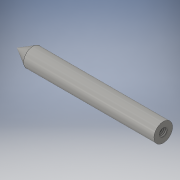
# Autodesk Inventor part: outerTubeStopPost
Saved by Autodesk Inventor 2016 SP1 (Build 200210100, 210)
## iProperties
Created: 2016-02-17
Part Number: outerTubeStopPost
Material: Steel
Document SubType Name: Modeling
Designer: steele
Density: 7.85 g/cm^3
Appearance: Plate
Mass: 46.6508 g
Surface Area: 26.2714 cm^2
Volume: 5.94278 cm^3
Author: steele
Autodesk Inventor part; units mm, degrees
ref_plane "YZ Plane" through (0, 0, 0) normal (1, 0, 0) x (0, 1, 0)
ref_plane "XZ Plane" through (0, 0, 0) normal (0, 1, 0) x (-1, 0, 0)
ref_plane "XY Plane" through (0, 0, 0) normal (0, 0, 1) x (1, 0, 0)
sketch "Sketch1" plane through (0, 0, 0) normal (1, 0, 0) x (0, 1, 0)
  circle A0 centre (0, 0) radius 4.7625
  dimension "d0" = 9.525
  constraints: 1 centre point, 1 coincident
  measures "d0" diameter of A0
extrude "Extrusion1" add sketch "Sketch1" along normal mid plane 74.93
sketch "Sketch2" plane through (0, 0, 0) normal (0, 1, 0) x (-1, 0, 0)
  line L0 (37.465, -4.7625) -> (37.465, 4.7625) projected
  line L1 (37.465, 0) -> (29.2161, -4.7625)
  line L2 (37.465, -4.7625) -> (-37.465, -4.7625) projected
  line L3 (37.465, -4.7625) -> (37.465, 0)
  line L4 (50.2285, 0) -> (-50.2285, 0) projected
  point P0 (0, 0)
  dimension "d3" = 60
  dimension "d5" = 8.2489
  constraints: 4 end point, 1 collinear, 1 midpoint, 1 point on line
  measures "d3" angle of L0 L1
  measures "d5" distance of L1.end L0.start
revolve "Revolution1" cut sketch "Sketch2" angle 360 about axis through (-10, 0, 0) along (1, 0, 0)
sketch "Sketch3" plane through (37.465, 0, 0) normal (1, 0, 0) x (0, 0, -1)
  point P0 (0, 0)
  point P1 (0, 0)
  constraints: 1 coincident
hole "Hole1" at (37.465, 0, 0) direction (-1, 0, 0) diameter 3.9624 depth 12.7 tip angle 118 thread size "10-32 UNF" class "2B" standard "ANSI Unified Screw Threads"
equation "\"d0\" = diam"
equation "\"d1\" = length"
equation "\"diam\" = 9.525"
equation "\"nosePiece_drivenDimesion\" = 8.255"
equation "\"spacerFromOuterTube\" = 3.175"
equation "\"length\" = 74.93"
body "Solid1"
